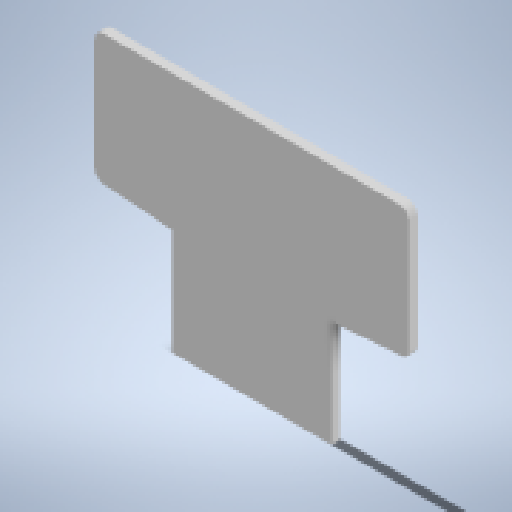
# Autodesk Inventor part: top_enclosure
Saved by Autodesk Inventor 2023.3 (Build 273359000, 359)
## iProperties
Created: 2023-12-09
Part Number: top_enclosure
Material: Generic
Document SubType Name: Modeling
Designer: mmelin
Density: 1 g/cm^3
Appearance: Default
Author: mmelin
Autodesk Inventor part; units mm, degrees
ref_plane "YZ Plane" through (0, 0, 0) normal (1, 0, 0) x (0, 1, 0)
ref_plane "XZ Plane" through (0, 0, 0) normal (0, 1, 0) x (-1, 0, 0)
ref_plane "XY Plane" through (0, 0, 0) normal (0, 0, 1) x (1, 0, 0)
sketch "Sketch1" plane through (0, 0, 0) normal (0, 0, 1) x (1, 0, 0)
  line L0 (-2.75, 3.25) -> (-4.7407, 3.4125) projected
  arc A0 (-5.2, 3.9108) -> (-4.7407, 3.4125) centre (-4.7, 3.9108) ccw projected
  line L1 (-5.2, 3.9108) -> (-5.2, 7.45) projected
  arc A1 (-4.7, 7.95) -> (-5.2, 7.45) centre (-4.7, 7.45) ccw projected
  arc A2 (5.2176, 3.2181) -> (5.6, 3.45) centre (5.1769, 3.7165) ccw projected
  line L2 (5.6, 3.45) -> (5.6, 7.75) projected
  arc A3 (5.6, 7.75) -> (5.1, 8.25) centre (5.1, 7.75) ccw projected
  line L3 (-5.1, 8.25) -> (5.1, 8.25) projected
  arc A4 (-5.1, 8.25) -> (-5.6, 7.75) centre (-5.1, 7.75) ccw projected
  line L4 (-5.6, 3.45) -> (-5.6, 7.75) projected
  arc A5 (-5.6, 3.45) -> (-5.2176, 3.2181) centre (-5.1769, 3.7165) ccw projected
  line L5 (-5.2176, 3.2181) -> (-3.1663, 3.0507) projected
  arc A6 (-3.15, 2.7961) -> (-3.1663, 3.0507) centre (-5.15, 2.7961) ccw projected
  line L6 (-3.15, -0.45) -> (-3.15, 2.7961) projected
  line L7 (3.15, -0.45) -> (-3.15, -0.45) projected
  line L8 (3.15, 2.7961) -> (3.15, -0.45) projected
  arc A7 (3.1663, 3.0507) -> (3.15, 2.7961) centre (5.15, 2.7961) ccw projected
  line L9 (3.1663, 3.0507) -> (5.2176, 3.2181) projected
  line L10 (2.75, -0.15) -> (2.75, 3.25) projected
  line L11 (-2.75, -0.15) -> (2.75, -0.15) projected
  line L12 (-2.75, 3.25) -> (-2.75, -0.15) projected
  line L13 (-2.75, 3.25) -> (-4.7407, 3.4125) projected
  arc A8 (-5.2, 3.9108) -> (-4.7407, 3.4125) centre (-4.7, 3.9108) ccw projected
  line L14 (-5.2, 3.9108) -> (-5.2, 7.45) projected
  arc A9 (-4.7, 7.95) -> (-5.2, 7.45) centre (-4.7, 7.45) ccw projected
  line L15 (-4.7, 7.95) -> (4.7, 7.95) projected
  arc A10 (5.2, 7.45) -> (4.7, 7.95) centre (4.7, 7.45) ccw projected
  line L16 (5.2, 3.9108) -> (5.2, 7.45) projected
  arc A11 (4.7407, 3.4125) -> (5.2, 3.9108) centre (4.7, 3.9108) ccw projected
  line L17 (4.7407, 3.4125) -> (2.75, 3.25) projected
  line L18 (-2.65, -0.05) -> (-2.65, 3.3422)
  line L19 (-2.65, 3.3422) -> (-4.7325, 3.5122)
  line L20 (-5.1, 3.9108) -> (-5.1, 7.45)
  line L21 (-4.7, 7.85) -> (4.7, 7.85)
  line L22 (5.1, 7.45) -> (5.1, 3.9108)
  line L23 (4.7325, 3.5122) -> (2.65, 3.3422)
  line L24 (2.65, 3.3422) -> (2.65, -0.05)
  line L25 (2.65, -0.05) -> (-2.65, -0.05)
  arc A12 (-5.1, 3.9108) -> (-4.7325, 3.5122) centre (-4.7, 3.9108) ccw
  arc A13 (4.7325, 3.5122) -> (5.1, 3.9108) centre (4.7, 3.9108) ccw
  arc A14 (-4.7, 7.85) -> (-5.1, 7.45) centre (-4.7, 7.45) ccw
  arc A15 (5.1, 7.45) -> (4.7, 7.85) centre (4.7, 7.45) ccw
  point P0 (0, 0)
  dimension "d0" = 0.1
  dimension "d1" = 0.1
  dimension "d2" = 0.1
  dimension "d3" = 0.1
  dimension "d4" = 0.1
  dimension "d5" = 0.1
  dimension "d6" = 0.1
  dimension "d7" = 0.1
  dimension "d8" = 0.4
  dimension "d9" = 0.4
  dimension "d10" = 0.4
  dimension "d11" = 0.4
  constraints: 16 end point, 9 parallel, 8 point on circle, 8 tangent, 4 centre point, 2 perpendicular, 1 horizontal
  measures "d0" distance between parallel lines of L11 L25
  measures "d1" distance between parallel lines of L12 L18
  measures "d2" distance between parallel lines of L10 L24
  measures "d3" distance between parallel lines of L15 L21
  measures "d4" distance between parallel lines of L1 L20
  measures "d5" distance between parallel lines of L16 L22
  measures "d6" distance between parallel lines of L0 L19
  measures "d7" distance between parallel lines of L17 L23
  measures "d8" radius of A12
  measures "d9" radius of A13
  measures "d10" radius of A14
  measures "d11" radius of A15
extrude "Extrusion1" add sketch "Sketch1" along normal blind 0.3 contours L18 L19 A12 L20 A14 L21 A15 L22 A13 L23 L24 L25
sketch "Sketch2" plane through (0, 0, 0.3) normal (0, 0, 1) x (1, 0, 0)
  line L0 (-2.35, 6.8) -> (0.15, 6.8)
  line L1 (0.15, 6.8) -> (0.15, 4.3)
  line L2 (0.15, 4.3) -> (-2.35, 4.3)
  line L3 (-2.35, 4.3) -> (-2.35, 6.8)
  line L4 (-5.1, 7.45) -> (-5.1, 3.9108) projected
  line L5 (4.7, 7.85) -> (-4.7, 7.85) projected
  point P0 (0, 0)
  dimension "d14" = 2.75
  dimension "d15" = 1.05
  dimension "d16" = 2.5
  dimension "d17" = 2.5
  constraints: 8 end point, 2 parallel, 1 horizontal, 1 perpendicular
  measures "d14" distance between parallel lines of L4 L3
  measures "d15" distance between parallel lines of L5 L0
  measures "d16" distance of L0.end L1.end
  measures "d17" distance of L1.end L2.end
extrude "Extrusion2" cut sketch "Sketch2" against normal blind 0.3
equation "\"d1\" = d0"
equation "\"d2\" = d0"
equation "\"d3\" = d0"
equation "\"d4\" = d0"
equation "\"d5\" = d0"
equation "\"d6\" = d0"
equation "\"d7\" = d0"
equation "\"d8\" = d10"
equation "\"d9\" = d10"
equation "\"d11\" = d10"
equation "\"d17\" = d16"
body "Solid1"
